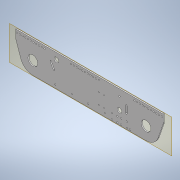
# Autodesk Inventor part: inside_plate
Saved by Autodesk Inventor 2022 (Build 260153000, 153)
## iProperties
Created: 2021-07-14
Part Number: inside_plate
Material: Generic
Document SubType Name: Modeling
Designer: gfellows
Density: 1 g/cm^3
Appearance: Default
Author: gfellows
Autodesk Inventor part; units mm, degrees
ref_plane "YZ Plane" through (0, 0, 0) normal (1, 0, 0) x (0, 1, 0)
ref_plane "XZ Plane" through (0, 0, 0) normal (0, 1, 0) x (-1, 0, 0)
ref_plane "XY Plane" through (0, 0, 0) normal (0, 0, 1) x (1, 0, 0)
ref_plane "Work Plane1" through (165.1, 7.35, 75.175) normal (0, 0, 1) x (1, 0, 0)
sketch "Sketch1" plane through (165.1, 7.35, 75.175) normal (0, 0, 1) x (1, 0, 0)
  circle A0 centre (165.1, -7.35) radius 14.2748 projected
  circle A1 centre (-165.1, -7.35) radius 14.2748 projected
  circle A2 centre (87.5541, -7.15) radius 7.008 projected
  circle A3 centre (-96.2421, 28.6508) radius 7.008 projected
  line L0 (59.5541, -26.1492) -> (-64.3229, -26.1492) construction
  line L1 (-64.3229, 11.8492) -> (59.5541, 11.8492) construction
  line L2 (-64.3229, -26.1492) -> (-64.3229, 11.8492) construction
  line L3 (59.5541, 11.8492) -> (59.5541, -26.1492) construction
  line L4 (73.4511, 2.35) -> (73.4511, -16.65) construction
  line L5 (59.5541, 2.35) -> (73.4511, 2.35) construction
  line L6 (73.4511, -16.65) -> (59.5541, -16.65) construction
  line L7 (112.5541, -44.65) -> (88.5541, -44.65) construction
  line L8 (88.5541, -44.65) -> (88.5541, -20.65) construction
  line L9 (85.5541, -20.65) -> (85.5541, -44.65) construction
  line L10 (85.5541, -44.65) -> (61.5541, -44.65) construction
  line L11 (61.5541, -44.65) -> (61.5541, -20.65) construction
  line L12 (61.5541, -20.65) -> (85.5541, -20.65) construction
  line L13 (88.5541, -20.65) -> (112.5541, -20.65) construction
  line L14 (112.5541, -20.65) -> (112.5541, -44.65) construction
  arc A4 (56.5541, -44.65) -> (60.5541, -40.65) centre (56.5541, -40.65) ccw construction
  arc A5 (-200.3988, -19.4033) -> (-165.1, -44.65) centre (-165.1, -7.35) ccw projected
  line L15 (215.1, 47.65) -> (-215.1, 47.65) projected
  arc A6 (165.1, -44.65) -> (200.3988, -19.4033) centre (165.1, -7.35) ccw projected
  arc A7 (113.5541, -40.65) -> (117.5541, -44.65) centre (117.5541, -40.65) ccw construction
  line L16 (113.5541, -23.65) -> (113.5541, -40.65) construction
  arc A8 (113.5541, -23.65) -> (109.5541, -19.65) centre (109.5541, -23.65) ccw construction
  line L17 (64.5541, -19.65) -> (109.5541, -19.65) construction
  arc A9 (64.5541, -19.65) -> (60.5541, -23.65) centre (64.5541, -23.65) ccw construction
  line L18 (60.5541, -40.65) -> (60.5541, -23.65) construction
  circle A10 centre (-165.1, -7.35) radius 14.2748 projected
  circle A11 centre (165.1, -7.35) radius 14.2748 projected
  circle A12 centre (-96.2421, 28.6508) radius 7.008 projected
  circle A13 centre (87.5541, -7.15) radius 7.008 projected
  line L19 (56.5541, -44.65) -> (117.5541, -44.65)
  circle A14 centre (65.5541, -24.65) radius 2
  circle A15 centre (81.5541, -24.65) radius 2
  circle A16 centre (65.5541, -40.65) radius 2
  circle A17 centre (81.5541, -40.65) radius 2
  circle A18 centre (92.5541, -24.65) radius 2
  circle A19 centre (108.5541, -24.65) radius 2
  circle A20 centre (108.5541, -40.65) radius 2
  circle A21 centre (92.5541, -40.65) radius 2
  circle A22 centre (27.1666, 8.85) radius 1.3526
  circle A23 centre (43.1665, 8.85) radius 1.3526
  circle A24 centre (27.1666, -23.15) radius 1.3526
  circle A25 centre (43.1665, -23.15) radius 1.3526
  line L20 (27.1666, 8.85) -> (43.1665, -23.15) construction
  line L21 (73.4511, -7.15) -> (-64.3229, -7.15) construction
  line L22 (-165.1, -44.65) -> (56.5541, -44.65) projected
  line L23 (-214.6708, 22.3931) -> (-200.3988, -19.4033) projected
  line L24 (-215.1, 47.65) -> (-215.1, 24.9782) projected
  line L25 (200.3988, -19.4033) -> (214.6708, 22.3931) projected
  line L26 (117.5541, -44.65) -> (165.1, -44.65) projected
  arc A26 (214.6708, 22.3931) -> (215.1, 24.9782) centre (207.1, 24.9782) ccw projected
  arc A27 (-215.1, 24.9782) -> (-214.6708, 22.3931) centre (-207.1, 24.9782) ccw projected
  circle A28 centre (-4.9, 39.65) radius 2 projected
  line L27 (31.1, 47.65) -> (31.1, 35.65) projected
  line L28 (-56.9, 47.65) -> (31.1, 47.65) projected
  line L29 (-56.9, 47.65) -> (-56.9, 35.65) projected
  line L30 (-56.9, 35.65) -> (31.1, 35.65) projected
  circle A29 centre (11.1, 39.65) radius 2 projected
  circle A30 centre (3.1, 39.65) radius 2 projected
  circle A31 centre (-4.9, 39.65) radius 2 projected
  circle A32 centre (-12.9, 39.65) radius 2 projected
  circle A33 centre (-20.9, 39.65) radius 2 projected
  circle A34 centre (-28.9, 39.65) radius 2 projected
  circle A35 centre (-36.9, 39.65) radius 2 projected
  circle A36 centre (-44.9, 39.65) radius 2 projected
  circle A37 centre (-52.9, 39.65) radius 2 projected
  circle A38 centre (19.1, 39.65) radius 2 projected
  circle A39 centre (27.1, 39.65) radius 2 projected
  line L31 (-215.1, 45.15) -> (-127.1, 45.15) projected
  line L32 (-127.1, 47.65) -> (-127.1, 35.65) projected
  line L33 (-215.1, 47.65) -> (-127.1, 47.65) projected
  line L34 (-215.1, 47.65) -> (-215.1, 35.65) projected
  line L35 (-215.1, 35.65) -> (-127.1, 35.65) projected
  circle A40 centre (-147.1, 39.65) radius 2 projected
  circle A41 centre (-155.1, 39.65) radius 2 projected
  circle A42 centre (-163.1, 39.65) radius 2 projected
  circle A43 centre (-171.1, 39.65) radius 2 projected
  circle A44 centre (-179.1, 39.65) radius 2 projected
  circle A45 centre (-187.1, 39.65) radius 2 projected
  circle A46 centre (-195.1, 39.65) radius 2 projected
  circle A47 centre (-203.1, 39.65) radius 2 projected
  circle A48 centre (-211.1, 39.65) radius 2 projected
  circle A49 centre (-139.1, 39.65) radius 2 projected
  circle A50 centre (-131.1, 39.65) radius 2 projected
  line L36 (215.1, 47.65) -> (215.1, 35.65) projected
  line L37 (127.1, 47.65) -> (215.1, 47.65) projected
  line L38 (127.1, 47.65) -> (127.1, 35.65) projected
  line L39 (127.1, 35.65) -> (215.1, 35.65) projected
  circle A51 centre (195.1, 39.65) radius 2 projected
  circle A52 centre (187.1, 39.65) radius 2 projected
  circle A53 centre (179.1, 39.65) radius 2 projected
  circle A54 centre (171.1, 39.65) radius 2 projected
  circle A55 centre (163.1, 39.65) radius 2 projected
  circle A56 centre (155.1, 39.65) radius 2 projected
  circle A57 centre (147.1, 39.65) radius 2 projected
  circle A58 centre (139.1, 39.65) radius 2 projected
  circle A59 centre (131.1, 39.65) radius 2 projected
  circle A60 centre (203.1, 39.65) radius 2 projected
  circle A61 centre (211.1, 39.65) radius 2 projected
  line L40 (215.1, 24.9782) -> (215.1, 47.65) projected
  arc A62 (109.5868, 15.55) -> (105.5868, 15.55) centre (107.5868, 15.55) ccw projected
  line L41 (105.5868, -4.45) -> (105.5868, 15.55) projected
  arc A63 (105.5868, -4.45) -> (109.5868, -4.45) centre (107.5868, -4.45) ccw projected
  line L42 (109.5868, 15.55) -> (109.5868, -4.45) projected
  arc A64 (-105.2208, -1.6588) -> (-101.6761, 0.1945) centre (-103.4484, -0.7322) ccw projected
  line L43 (-110.9425, 17.9183) -> (-101.6761, 0.1945) projected
  arc A65 (-110.9425, 17.9183) -> (-114.4873, 16.065) centre (-112.7149, 16.9916) ccw projected
  line L44 (-105.2208, -1.6588) -> (-114.4873, 16.065) projected
  circle A66 centre (-139.1, 39.65) radius 2 projected
  circle A67 centre (-155.1, 39.65) radius 2 projected
  circle A68 centre (-179.1, 39.65) radius 2 projected
  circle A69 centre (-187.1, 39.65) radius 2 projected
  circle A70 centre (-203.1, 39.65) radius 2 projected
  circle A71 centre (211.1, 39.65) radius 2 projected
  circle A72 centre (195.1, 39.65) radius 2 projected
  circle A73 centre (179.1, 39.65) radius 2 projected
  circle A74 centre (163.1, 39.65) radius 2 projected
  circle A75 centre (131.1, 39.65) radius 2 projected
  circle A76 centre (139.1, 39.65) radius 2 projected
  circle A77 centre (147.1, 39.65) radius 2 projected
  circle A78 centre (155.1, 39.65) radius 2 projected
  circle A79 centre (171.1, 39.65) radius 2 projected
  circle A80 centre (187.1, 39.65) radius 2 projected
  circle A81 centre (203.1, 39.65) radius 2 projected
  circle A82 centre (-211.1, 39.65) radius 2 projected
  circle A83 centre (-195.1, 39.65) radius 2 projected
  circle A84 centre (-171.1, 39.65) radius 2 projected
  circle A85 centre (-163.1, 39.65) radius 2 projected
  circle A86 centre (-147.1, 39.65) radius 2 projected
  circle A87 centre (-131.1, 39.65) radius 2 projected
  circle A88 centre (87.5541, 28.6508) radius 2 projected
  circle A89 centre (-99.4459, -35.3996) radius 2 projected
  circle A90 centre (-51.4459, -35.3996) radius 2 projected
  circle A91 centre (-3.4459, -35.3996) radius 2 projected
  circle A92 centre (44.5541, -35.3996) radius 2 projected
  circle A93 centre (118.5541, -39.65) radius 2 projected
  point P0 (35.1666, -7.15)
  point P1 (207.1, 24.9782)
  dimension "d2" = 4
  dimension "d5" = 16
  dimension "d8" = 16
  dimension "d11" = 4
  dimension "d12" = 4
  dimension "d15" = 27
  dimension "d20" = 2.7051
  dimension "d23" = 16
  dimension "d30" = 31.9999
  dimension "d35" = 52.3875
  constraints: 12 centre point, 6 end point, 4 horizontal, 3 midpoint, 2 vertical, 1 point on line, 1 tangent, 20 other
  measures "d2" diameter of A14
  measures "d5" distance of A14.centre A15.centre
  measures "d8" distance of A14.centre A16.centre
  measures "d11" distance from line of L12 A14.centre
  measures "d12" distance from line of L11 A14.centre
  measures "d15" distance of A14.centre A18.centre
  measures "d20" diameter of A22
  measures "d23" distance of L20.start A23.centre
  measures "d30" distance of L20.start A24.centre
  measures "d35" distance of A2.centre point (35.167, -7.15)
extrude "Extrusion1" add sketch "Sketch1" along normal blind 3.175
body "Solid1"
